Autodesk Fusion 360 part; units mm, degrees
(part 4 of 4)
  spline S218 degree 3 poles (2.5124, -1.7393) (1.6846, -2.1155) (0.8323, -2.1832) (-0.0445, -1.9423) knots 0 0 0 0 1 1 1 1
  spline S219 degree 3 poles (-0.0445, -1.9423) (-0.2359, -1.86) (-0.3982, -1.7382) (-0.5316, -1.577) knots 0 0 0 0 1 1 1 1
  spline S220 degree 3 poles (-0.5316, -1.577) (-0.5586, -1.5499) (-0.5857, -1.5499) (-0.6127, -1.577) knots 0 0 0 0 1 1 1 1
  spline S221 degree 3 poles (-0.6127, -1.577) (-1.2648, -2.4997) (-1.948, -3.3993) (-2.6623, -4.2759) knots 0 0 0 0 1 1 1 1
  spline S222 degree 3 poles (-2.6623, -4.2759) (-2.9289, -4.5697) (-3.2198, -4.8336) (-3.5349, -5.0674) knots 0 0 0 0 1 1 1 1
  spline S223 degree 3 poles (-3.5349, -5.0674) (-4.2399, -5.1741) (-4.5443, -4.8697) (-4.4481, -4.1542) knots 0 0 0 0 1 1 1 1
  spline S224 degree 3 poles (-4.4481, -4.1542) (-4.3995, -3.9625) (-4.3184, -3.7866) (-4.2046, -3.6266) knots 0 0 0 0 1 1 1 1
  spline S225 degree 3 poles (-4.2046, -3.6266) (-3.7014, -3.0014) (-3.1534, -2.4129) (-2.5608, -1.8611) knots 0 0 0 0 1 1 1 1
  spline S226 degree 3 poles (-2.5608, -1.8611) (-1.8926, -1.2876) (-1.2365, -0.6991) (-0.5924, -0.0956) knots 0 0 0 0 1 1 1 1
  spline S227 degree 3 poles (-0.5924, -0.0956) (-0.1256, 0.5672) (0.3006, 1.2571) (0.686, 1.9743) knots 0 0 0 0 1 1 1 1
  spline S228 degree 3 poles (0.686, 1.9743) (0.4059, 2.0036) (0.1353, 1.9562) (-0.1257, 1.8322) knots 0 0 0 0 1 1 1 1
  spline S229 degree 3 poles (-0.1257, 1.8322) (-1.0853, 1.3734) (-1.9173, 0.7443) (-2.6217, -0.055) knots 0 0 0 0 1 1 1 1
  spline S230 degree 3 poles (-2.6217, -0.055) (-2.9798, -0.5006) (-3.318, -0.9605) (-3.6364, -1.4349) knots 0 0 0 0 1 1 1 1
  spline S231 degree 3 poles (-3.6364, -1.4349) (-3.6067, -1.6426) (-3.5729, -1.8522) (-3.5349, -2.064) knots 0 0 0 0 1 1 1 1
  spline S232 degree 3 poles (-3.5349, -2.064) (-3.5595, -2.4471) (-3.7624, -2.6704) (-4.1437, -2.7337) knots 0 0 0 0 1 1 1 1
  spline S233 degree 3 poles (-4.1437, -2.7337) (-4.4659, -2.7158) (-4.6756, -2.5535) (-4.7728, -2.2467) knots 0 0 0 0 1 1 1 1
  spline S234 degree 3 poles (-4.7728, -2.2467) (-4.784, -2.0854) (-4.7908, -1.9298) (-4.7931, -1.7799) knots 0 0 0 0 1 1 1 1
  spline S235 degree 3 poles (-4.7931, -1.7799) (-5.1055, -1.746) (-5.4167, -1.7054) (-5.7265, -1.6582) knots 0 0 0 0 1 1 1 1
  spline S236 degree 3 poles (-5.7265, -1.6582) (-6.0883, -1.5099) (-6.2166, -1.2461) (-6.1123, -0.8667) knots 0 0 0 0 1 1 1 1
  spline S237 degree 3 poles (-6.1123, -0.8667) (-6.0692, -0.7402) (-6.0149, -0.6184) (-5.9499, -0.5015) knots 0 0 0 0 1 1 1 1
  spline S238 degree 3 poles (-5.9499, -0.5015) (-5.6485, -0.0748) (-5.3373, 0.3445) (-5.0163, 0.7567) knots 0 0 0 0 1 1 1 1
  spline S239 degree 3 poles (-5.0163, 0.7567) (-4.7945, 1.0603) (-4.6051, 1.385) (-4.4481, 1.7308) knots 0 0 0 0 1 1 1 1
  spline S240 degree 3 poles (-4.4481, 1.7308) (-4.382, 1.9045) (-4.3752, 2.0804) (-4.4278, 2.2584) knots 0 0 0 0 1 1 1 1
  spline S241 degree 3 poles (-4.4278, 2.2584) (-4.4862, 2.2812) (-4.5471, 2.2948) (-4.6104, 2.299) knots 0 0 0 0 1 1 1 1
  spline S242 degree 3 poles (-4.6104, 2.299) (-5.4737, 2.0991) (-6.2787, 1.7609) (-7.0254, 1.2843) knots 0 0 0 0 1 1 1 1
  spline S243 degree 3 poles (-7.0254, 1.2843) (-7.1253, 0.7409) (-7.3282, 0.2404) (-7.6342, -0.2174) knots 0 0 0 0 1 1 1 1
  spline S244 degree 3 poles (-7.6342, -0.2174) (-7.4163, -0.5815) (-7.5109, -0.825) (-7.9183, -0.9479) knots 0 0 0 0 1 1 1 1
  spline S245 degree 3 poles (-7.9183, -0.9479) (-8.0068, -0.9441) (-8.088, -0.917) (-8.1619, -0.8667) knots 0 0 0 0 1 1 1 1
  spline S246 degree 3 poles (-8.1619, -0.8667) (-8.7353, -1.4174) (-9.3847, -1.8571) (-10.11, -2.1858) knots 0 0 0 0 1 1 1 1
  spline S247 degree 3 poles (-10.11, -2.1858) (-10.7857, -2.4482) (-11.4489, -2.4212) (-12.0987, -2.1046) knots 0 0 0 0 1 1 1 1
  spline S248 degree 3 poles (-12.0987, -2.1046) (-12.7566, -1.5763) (-12.8446, -0.9608) (-12.3625, -0.258) knots 0 0 0 0 1 1 1 1
  spline S249 degree 3 poles (-12.3625, -0.258) (-11.7805, 0.2999) (-11.084, 0.584) (-10.2723, 0.5943) knots 0 0 0 0 1 1 1 1
  spline S250 degree 3 poles (-10.2723, 0.5943) (-9.6221, 0.5586) (-8.993, 0.4234) (-8.3851, 0.1885) knots 0 0 0 0 1 1 1 1
  spline S251 degree 3 poles (-8.3851, 0.1885) (-8.0888, 0.5449) (-7.9196, 0.9575) (-7.8777, 1.4264) knots 0 0 0 0 1 1 1 1
  spline S252 degree 3 poles (-7.8777, 1.4264) (-7.8928, 1.6325) (-7.9739, 1.8084) (-8.1213, 1.954) knots 0 0 0 0 1 1 1 1
  spline S253 degree 3 poles (-8.1213, 1.954) (-8.2438, 1.9594) (-8.3522, 2) (-8.446, 2.0757) knots 0 0 0 0 1 1 1 1
  spline S254 degree 3 poles (-8.446, 2.0757) (-8.9366, 2.1144) (-9.4237, 2.0873) (-9.907, 1.9946) knots 0 0 0 0 1 1 1 1
  spline S255 degree 3 poles (-9.907, 1.9946) (-11.0333, 1.6547) (-12.0479, 1.1136) (-12.951, 0.3711) knots 0 0 0 0 1 1 1 1
  spline S256 degree 3 poles (-12.951, 0.3711) (-13.7099, -0.5701) (-14.6434, -1.2872) (-15.7514, -1.7799) knots 0 0 0 0 1 1 1 1
  spline S257 degree 3 poles (-15.7514, -1.7799) (-16.4036, -2.0727) (-17.0798, -2.1539) (-17.7807, -2.0234) knots 0 0 0 0 1 1 1 1
  spline S258 degree 3 poles (-17.7807, -2.0234) (-18.5116, -1.861) (-18.8834, -1.4079) (-18.8968, -0.6638) knots 0 0 0 0 1 1 1 1
  spline S259 degree 3 poles (-18.8968, -0.6638) (-19.0583, -0.836) (-19.2543, -0.9104) (-19.4853, -0.887) knots 0 0 0 0 1 1 1 1
  spline S260 degree 3 poles (-19.4853, -0.887) (-19.7568, -0.7823) (-19.8445, -0.5861) (-19.7491, -0.2985) knots 0 0 0 0 1 1 1 1
  spline S261 degree 3 poles (-19.7491, -0.2985) (-18.9755, 0.2043) (-18.2247, 0.7387) (-17.4966, 1.3046) knots 0 0 0 0 1 1 1 1
  spline S262 degree 3 poles (-17.4966, 1.3046) (-17.2742, 1.4862) (-17.098, 1.7027) (-16.969, 1.954) knots 0 0 0 0 1 1 1 1
  spline S263 degree 3 poles (-16.969, 1.954) (-16.9856, 1.9923) (-17.0124, 2.0194) (-17.0501, 2.0351) knots 0 0 0 0 1 1 1 1
  spline S264 degree 3 poles (-17.0501, 2.0351) (-17.4162, 2.0756) (-17.7681, 2.0214) (-18.1054, 1.8728) knots 0 0 0 0 1 1 1 1
  spline S265 degree 3 poles (-18.1054, 1.8728) (-19.0867, 1.4199) (-19.9187, 0.7772) (-20.6014, -0.055) knots 0 0 0 0 1 1 1 1
  spline S266 degree 3 poles (-20.6014, -0.055) (-20.9322, -0.4461) (-21.2232, -0.8655) (-21.474, -1.3132) knots 0 0 0 0 1 1 1 1
  spline S267 degree 3 poles (-21.474, -1.3132) (-21.2869, -1.7955) (-21.4492, -2.0187) (-21.961, -1.9828) knots 0 0 0 0 1 1 1 1
  spline S268 degree 3 poles (-21.961, -1.9828) (-22.2788, -1.7875) (-22.4006, -1.5102) (-22.3263, -1.1508) knots 0 0 0 0 1 1 1 1
  spline S269 degree 3 poles (-22.3263, -1.1508) (-22.9895, -1.6347) (-23.7269, -1.9323) (-24.5382, -2.0437) knots 0 0 0 0 1 1 1 1
  spline S270 degree 3 poles (-24.5382, -2.0437) (-25.1437, -2.0526) (-25.5159, -1.7685) (-25.6543, -1.1914) knots 0 0 0 0 1 1 1 1
  spline S271 degree 3 poles (-25.6543, -1.1914) (-25.6413, -1.0535) (-25.6547, -0.9182) (-25.6949, -0.7856) knots -1 -1 -1 -1 0 0 0 0
  spline S272 degree 3 poles (-25.6949, -0.7856) (-25.7197, -0.7906) (-25.7331, -0.8041) (-25.7355, -0.8262) knots -1 -1 -1 -1 0 0 0 0
  line L59 (-31.5258, -3.8371) -> (-34.2, -5.2) construction
  line L60 (-34.2, -5.2) -> (-36.3369, -2.9858) construction
  spline S273 degree 2 poles (-31.5258, -3.8371) (-34.2, -5.2) (-36.3369, -2.9858) knots 0 0 0 1 1 1
  line L61 (-30.7373, 5.7363) -> (-33.3647, 7.7826) construction
  line L62 (-33.3647, 7.7826) -> (-36.3369, 4.9858) construction
  spline S274 degree 2 poles (-30.7373, 5.7363) (-33.3647, 7.7826) (-36.3369, 4.9858) knots 0 0 0 1 1 1
  constraint coincident A0 L60.end
  constraint coincident A0 L62.end
extrude "Extrude4" add sketch "Sketch3" against normal blind 2.5 contours S0 S1 S2 A0 S273 | S82 A0 S274 bodies 1
sketch "Sketch4" plane through (0, 0, 0) normal (0, 0, 1) x (-1, 0, 0)
  circle A0 centre (-35, 1) radius 2.5
  dimension "d10" = 5
  measures "d10" diameter of A0
extrude "Extrude5" cut sketch "Sketch4" against normal blind 4.5 bodies 1
copy_body "Body->Comp1" bodies 1 removing the originals makes body 2 in component "Keyring"
component "Keyring" placed x (1, 0, 0) y (0, 1, 0) z (0, 0, 1) at (0, 0, 0)
named bodies: "Keyring"
